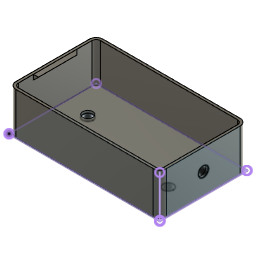
Template Box Fusion360 (Autodesk Fusion 360 design; units mm, degrees)
Autodesk Fusion 360 part; units mm, degrees
note: some values were not read from the file. Set by a fixed rule: which face or edge a step refers to.
sketch "Base" plane through (0, 0, 0) normal (0, 1, 0) x (1, 0, 0) in component "Top"
  line L0 (0, 0) -> (90, 0)
  line L1 (90, 0) -> (90, 52)
  line L2 (90, 52) -> (0, 52)
  line L3 (0, 52) -> (0, 0)
  dimension "d6" = 90
  dimension "d7" = 52
  constraint horizontal L0
  constraint vertical L1
  constraint horizontal L2
  constraint vertical L3
  constraint coincident L0.start L3.end
  measures "d6" distance of L0.start L0.end
  measures "d7" distance of L0.start L2.end
extrude "Extrude1" add sketch "Base" along normal blind 25 makes body 1 in component "Top"
fillet "Fillet1" radius 4 4 edges at (90, 12.5, 0) (0, 12.5, 0) (90, 12.5, -52) (0, 12.5, -52) on bodies 1 in component "Top"
shell "Shell1" thickness 1.5 removed faces 1 at (58.6667, 25, -17.3333) on bodies 1 in component "Top"
sketch "Knob" plane through (1.5, 0, 0) normal (1, 0, 0) x (0, 0, -1) in component "Top"
  line L0 (48, 1.5) -> (48, 25)
  line L1 (48, 25) -> (4, 25)
  line L2 (4, 25) -> (4, 1.5)
  line L3 (4, 1.5) -> (48, 1.5)
  line L4 (13, 25) -> (39, 25)
  line L5 (39, 25) -> (39, 22)
  line L6 (39, 22) -> (13, 22)
  line L7 (13, 22) -> (13, 25)
  line L8 (26, 25) -> (26, 22) construction
  dimension "d12" = 26
  dimension "d13" = 3
  constraint horizontal L4
  constraint vertical L5
  constraint horizontal L6
  constraint vertical L7
  constraint coincident L1 L4.start
  constraint midpoint L1 L8.start
  constraint midpoint L6 L8.end
  constraint vertical L8
  measures "d12" distance of L5.end L6.end
  measures "d13" distance of L4.end L5.end
extrude "Extrude2" add sketch "Knob" along normal blind 6 draft -45 contours L1 L4 L5 L6 L7 bodies 1 in component "Top"
ref_plane "WorkPlane2" through (45, 12.5, -26) normal (-1, 0, 0) x (0, 0, 1) in component "Top"
mirror "Mirror1" about plane through (45, 12.5, -26) normal (-1, 0, 0) of "Extrude2" in component "Top"
sketch "Top" plane through (0, 25, 0) normal (0, 1, 0) x (-1, 0, 0) in component "Base"
  line L0 (-90, -4) -> (-90, -48)
  arc A0 (-90, -48) -> (-86, -52) centre (-86, -48) ccw
  line L1 (-86, -52) -> (-4, -52)
  arc A1 (-4, -52) -> (0, -48) centre (-4, -48) ccw
  line L2 (0, -48) -> (0, -4)
  arc A2 (0, -4) -> (-4, 0) centre (-4, -4) ccw
  line L3 (-4, 0) -> (-86, 0)
  arc A3 (-86, 0) -> (-90, -4) centre (-86, -4) ccw
  line L4 (-88.5, -13) -> (-88.5, -4)
  arc A4 (-86, -1.5) -> (-88.5, -4) centre (-86, -4) ccw
  line L5 (-86, -1.5) -> (-4, -1.5)
  arc A5 (-1.5, -4) -> (-4, -1.5) centre (-4, -4) ccw
  line L6 (-1.5, -4) -> (-1.5, -13)
  line L7 (-1.5, -13) -> (-1.5, -39)
  line L8 (-1.5, -39) -> (-1.5, -48)
  arc A6 (-4, -50.5) -> (-1.5, -48) centre (-4, -48) ccw
  line L9 (-4, -50.5) -> (-86, -50.5)
  arc A7 (-88.5, -48) -> (-86, -50.5) centre (-86, -48) ccw
  line L10 (-88.5, -48) -> (-88.5, -39)
  line L11 (-88.5, -39) -> (-88.5, -13)
extrude "Extrude1'" add sketch "Top" along normal blind 1.5 separate body contours L0 A0 L1 A1 L2 A2 L3 A3 | L4 A4 L5 A5 L6 L7 L8 A6 L9 A7 L10 L11 makes body 2 in component "Base"
sketch "Lip" plane through (0, 25, 0) normal (0, -1, 0) x (1, 0, 0) in component "Base"
  arc A0 (90, -4) -> (86, 0) centre (86, -4) ccw
  line L0 (86, 0) -> (4, 0)
  arc A1 (4, 0) -> (0, -4) centre (4, -4) ccw
  line L1 (0, -4) -> (0, -48)
  arc A2 (0, -48) -> (4, -52) centre (4, -48) ccw
  line L2 (4, -52) -> (86, -52)
  arc A3 (86, -52) -> (90, -48) centre (86, -48) ccw
  line L3 (90, -48) -> (90, -4)
  line L4 (88.3, -48) -> (88.3, -4)
  arc A4 (88.3, -4) -> (86, -1.7) centre (86, -4) ccw
  line L5 (86, -1.7) -> (4, -1.7)
  arc A5 (4, -1.7) -> (1.7, -4) centre (4, -4) ccw
  line L6 (1.7, -4) -> (1.7, -48)
  arc A6 (1.7, -48) -> (4, -50.3) centre (4, -48) ccw
  line L7 (4, -50.3) -> (86, -50.3)
  arc A7 (86, -50.3) -> (88.3, -48) centre (86, -48) ccw
  dimension "d19" = 1.7
extrude "Extrude2'" add sketch "Lip" along normal blind 3 contours L4 A4 L5 A5 L6 A6 L7 A7 bodies 2 in component "Base"
extrude "Extrude3" cut sketch "Knob" along normal blind 3 draft -45 from surface at 0.2 contours L1 L4 L5 L6 L7 bodies 2 in component "Base"
mirror "Mirror1'" about plane through (45, 12.5, -26) normal (-1, 0, 0) of "Extrude3" in component "Base"
shell "Shell1'" thickness 1.5 removed faces 1 at (59.4333, 22, -30.3333) on bodies 2 in component "Base"
chamfer "Chamfer1" distance 0.6 angle 45 2 edges at (1.7, 22, -26) (88.3, 22, -26) on bodies 2 in component "Base"
sketch "PCB Mount" plane through (0, 25, 0) normal (0, -1, 0) x (1, 0, 0) in component "Base"
  arc A0 (90, -4) -> (86, 0) centre (86, -4) ccw construction
  arc A1 (0, -48) -> (4, -52) centre (4, -48) ccw construction
  line L0 (88.8284, -1.1716) -> (1.1716, -50.8284) construction
  line L1 (67.5, -39) -> (22.5, -39)
  line L2 (22.5, -39) -> (22.5, -13)
  line L3 (22.5, -13) -> (67.5, -13)
  line L4 (67.5, -13) -> (67.5, -39)
  line L5 (67.5, -39) -> (22.5, -13) construction
  line L6 (22.5, -39) -> (67.5, -13) construction
  point P0 (45, -26)
  dimension "d33" = 45
  dimension "d34" = 26
  constraint midpoint A0 L0.start
  constraint midpoint A1 L0.end
  constraint perpendicular L1 L2
  constraint parallel L1 L3
  constraint parallel L2 L4
  constraint horizontal L1
  constraint coincident L5 P0
  constraint coincident L6 P0
  constraint midpoint L0 P0
  measures "d33" distance of L2.end L3.end
  measures "d34" distance of L1.end L2.end
extrude "Extrude5" add sketch "PCB Mount" along normal blind 3 bodies 2 in component "Base"
sketch "Right Holes" plane through (90, 0, 0) normal (1, 0, 0) x (0, 0, -1) in component "Top"
  line L0 (48, 25) -> (4, 25)
  line L1 (4, 25) -> (4, 0)
  line L2 (4, 0) -> (48, 0)
  line L3 (48, 0) -> (48, 25)
  circle A0 centre (26, 12.5) radius 3
  line L4 (0, 25) -> (0, 0)
  line L5 (0, 0) -> (52, 0)
  dimension "d41" = 6
  dimension "d42" = 26
  dimension "d43" = 12.5
  measures "d41" diameter of A0
  measures "d42" distance of A0.centre L4
  measures "d43" distance of A0.centre L5
extrude "Extrude3'" cut sketch "Right Holes" against normal up to surface (1.5 mm away) contours A0 bodies 1 in component "Top"
sketch "Top Holes" plane through (0, 0, 0) normal (0, 1, 0) x (1, 0, 0) in component "Top"
  circle A0 centre (15, 32) radius 3
  circle A1 centre (75, 20) radius 3
  line L0 (0, 52) -> (0, 0)
  line L1 (90, 52) -> (0, 52)
  line L2 (0, 0) -> (90, 0)
  line L3 (90, 0) -> (90, 52)
  dimension "d46" = 6
  dimension "d47" = 6
  dimension "d48" = 15
  dimension "d49" = 20
  dimension "d50" = 20
  dimension "d51" = 15
  measures "d46" diameter of A0
  measures "d47" diameter of A1
  measures "d48" distance of A0.centre L0
  measures "d49" distance of A0.centre L1
  measures "d50" distance of A1.centre L2
  measures "d51" distance of A1.centre L3
extrude "Extrude4" cut sketch "Top Holes" along normal up to surface (1.5 mm away) contours A0 | A1 bodies 1 in component "Top"
component "Enclosure" placed x (1, 0, 0) y (0, 1, 0) z (0, 0, 1) at (0, 0, 0)
component "Top" placed x (1, 0, 0) y (0, 1, 0) z (0, 0, 1) at (0, 0, 0) in component "Enclosure"
component "Base" placed x (1, 0, 0) y (0, 1, 0) z (0, 0, 1) at (0, 0, 0) in component "Enclosure"
equation "Length = 52 mm"
equation "Width = 90 mm"
equation "heigth = 25 mm"
equation "shell = 1.5 mm"
equation "gap = 0.2 mm"
equation "d6 = Width"
equation "d7 = Length"
equation "d8 = heigth"
equation "d11 = shell"
equation "d12 = Length / 2"
equation "d13 = shell * 2"
equation "d17 = shell"
equation "d19 = shell + gap"
equation "d20 = shell * 2"
equation "d23 = shell * 2"
equation "d26 = shell"
equation "d33 = Width / 2"
equation "d34 = Length / 2"
equation "d42 = Length / 2"
equation "d43 = heigth / 2"
